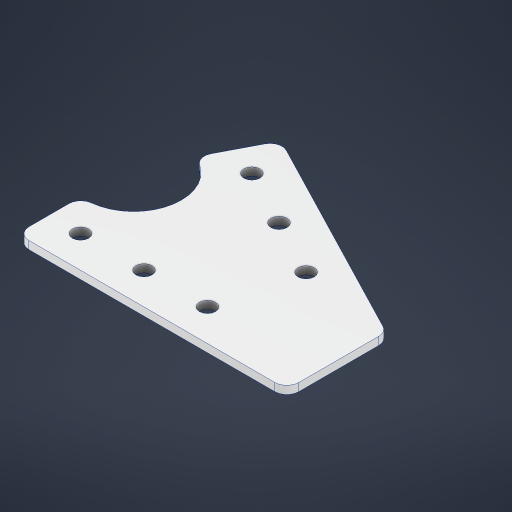
# Autodesk Inventor part: STRU_018_AngleBracket_62
Saved by Autodesk Inventor 2024.2 (Build 282272000, 272)
## iProperties
Created: 2024-07-25
Part Number: STRU_018_AngleBracket_62
Material: Aluminum 6061
Document SubType Name: Modeling
Designer: Bryan
Density: 2.7 g/cm^3
Appearance: Aluminum - Flat
Mass: 102.679 g
Surface Area: 149.238 cm^2
Volume: 38.0293 cm^3
Author: Bryan
Autodesk Inventor part; units mm, degrees
ref_plane "YZ Plane" through (0, 0, 0) normal (1, 0, 0) x (0, 1, 0)
ref_plane "XZ Plane" through (0, 0, 0) normal (0, 1, 0) x (-1, 0, 0)
ref_plane "XY Plane" through (0, 0, 0) normal (0, 0, 1) x (1, 0, 0)
sketch "Sketch1" plane through (0, 0, 0) normal (0, 1, 0) x (-1, 0, 0)
  line L0 (0, 0) -> (0, -39.7058)
  line L1 (0, 0) -> (107.95, 0)
  line L2 (107.95, 0) -> (107.95, -25.4)
  line L3 (107.95, -25.4) -> (27.5892, -25.4)
  line L4 (0, -39.7058) -> (87.2373, -84.9409)
  line L5 (0, -3.175) -> (38.1, -3.175) construction
  line L6 (38.1, -3.175) -> (38.1, -22.225) construction
  line L7 (38.1, -22.225) -> (0, -22.225) construction
  line L8 (0, -22.225) -> (0, -3.175) construction
  circle A0 centre (44.45, -12.7) radius 3.2512
  circle A1 centre (69.85, -12.7) radius 3.2512
  circle A2 centre (95.25, -12.7) radius 3.2512
  line L9 (27.5892, -25.4) -> (0, -18.6724) construction
  circle A3 centre (36.7113, -44.4359) radius 3.2512
  circle A4 centre (59.2601, -56.1281) radius 3.2512
  circle A5 centre (81.809, -67.8203) radius 3.2512
  line L10 (27.5892, -25.4) -> (98.9296, -62.392)
  line L11 (81.809, -67.8203) -> (93.0834, -73.6665) construction
  line L12 (98.9296, -62.392) -> (87.2373, -84.9409)
  point P0 (38.1, -12.7)
  dimension "d0" = 39.7058
  dimension "d1" = 25.4
  dimension "d2" = 27.5892
  dimension "d4" = 107.95
  dimension "d5" = 19.05
  dimension "d6" = 3.175
  dimension "d7" = 38.1
  dimension "d8" = 6.5024
  dimension "d9" = 6.35
  dimension "d10" = 25.4
  dimension "d11" = 25.4
  dimension "d14" = 62.592
  dimension "d15" = 12.7
  dimension "d16" = 27.408
  dimension "d17" = 166.296
  constraints: 27 end point, 6 centre point, 3 horizontal, 3 horizontal alignment, 3 parallel, 3 symmetric about line, 2 equal radius, 2 midpoint, 2 perpendicular, 2 point on line, 2 vertical, 3 other
  measures "d0" distance of L0.start L0.end
  measures "d1" distance of L1.end L2.end
  measures "d2" distance from line of L0 L3.end
  measures "d4" distance of L0.start L1.end
  measures "d5" distance of L5.end L6.end
  measures "d6" distance between parallel lines of L5 L1
  measures "d7" distance of L5.start L5.end
  measures "d8" diameter of A0
  measures "d9" distance from line of L6 A0.centre
  measures "d10" distance of A0.centre A1.centre
  measures "d11" distance of A1.centre A2.centre
  measures "d14" angle of L0 L10
  measures "d15" distance of L11.end L11.start
  measures "d16" angle of L10 L3
  measures "d17" angle of L10 L9
extrude "Extrusion1" add sketch "Sketch1" along normal blind 3.175
fillet "Fillet1" radius 19.05 1 edges at (-27.5892, 1.5875, -25.4)
fillet "Fillet2" radius 4.7625 6 edges at (-107.95, 1.5875, 0) (-107.95, 1.5875, -25.4) (-98.9296, 1.5875, -62.392) (-87.2373, 1.5875, -84.9409) (0, 1.5875, 0) (0, 1.5875, -39.7058)
body "Solid1"
